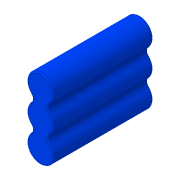
# Autodesk Inventor part: BatteryPack6600mAh
Saved by Autodesk Inventor 2017 (Build 210142000, 142)
## iProperties
Part Number: BatteryPack6600mAh
Material: Generisch
Document SubType Name: Modeling
Designer: Werkstatt
Density: 1 g/cm^3
Appearance: Vorgabe(1)
Author: Werkstatt
Autodesk Inventor part; units mm, degrees
ref_plane "YZ Plane" through (0, 0, 0) normal (1, 0, 0) x (0, 1, 0)
ref_plane "XZ Plane" through (0, 0, 0) normal (0, 1, 0) x (-1, 0, 0)
ref_plane "XY Plane" through (0, 0, 0) normal (0, 0, 1) x (1, 0, 0)
sketch "Skizze1" plane through (0, 0, 0) normal (0, 1, 0) x (-1, 0, 0)
  arc A0 (6.47, 11.83) -> (0, 27.45) centre (0, 18.3) ccw
  line L0 (9.15, 18.3) -> (9.15, 0) construction
  arc A1 (6.47, 11.83) -> (6.47, 6.47) centre (9.15, 9.15) ccw
  arc A2 (9.15, 0) -> (6.47, 6.47) centre (0, 0) ccw
  line L1 (0, 18.3) -> (0, 0) construction
  line L2 (0, 18.3) -> (0, 27.45) construction
  arc A3 (0, 27.45) -> (-6.47, 11.83) centre (0, 18.3) ccw
  arc A4 (-6.47, 6.47) -> (-6.47, 11.83) centre (-9.15, 9.15) ccw
  arc A5 (-6.47, 6.47) -> (-9.15, 0) centre (0, 0) ccw
  line L3 (9.15, 0) -> (-9.15, 0) construction
  line L4 (14.3464, 0) -> (-13.2665, 0) construction
  arc A6 (0, -27.45) -> (6.47, -11.83) centre (0, -18.3) ccw
  arc A7 (6.47, -6.47) -> (6.47, -11.83) centre (9.15, -9.15) ccw
  arc A8 (6.47, -6.47) -> (9.15, 0) centre (0, 0) ccw
  arc A9 (-6.47, -11.83) -> (-6.47, -6.47) centre (-9.15, -9.15) ccw
  arc A10 (-9.15, 0) -> (-6.47, -6.47) centre (0, 0) ccw
  arc A11 (-6.47, -11.83) -> (0, -27.45) centre (0, -18.3) ccw
  dimension "d1" = 18.3
  dimension "d3" = 9.15
  dimension "d5" = 9.15
  dimension "d6" = 9.15
  dimension "d7" = 9.15
  dimension "d8" = 3.79
  constraints: 25 point on circle, 12 centre point, 12 symmetric about line, 10 end point, 2 horizontal, 2 vertical, 1 coincident, 1 midpoint, 9 other
  measures "d1" distance of point (0, 0) L1.start
  measures "d3" horizontal distance of point (0, 0) A1.centre
  measures "d5" radius of A2
  measures "d6" radius of A0
  measures "d7" horizontal distance of point (0, 0) A1.centre
  measures "d8" radius of A1
extrude "Extrusion1" add sketch "Skizze1" along normal blind 69
fillet "Rundung1" radius 1 16 edges at (5.3599, 69, 9.15) (8.4535, 69, -3.5016) (5.3599, 69, -9.15) (-8.4535, 69, -21.8016) (-5.3599, 69, -9.15) (-8.4535, 69, 3.5016) (-5.3599, 69, 9.15) (8.4535, 69, 21.8016) (5.3599, 0, 9.15) (8.4535, 0, 3.5016) (5.3599, 0, -9.15) (-8.4535, 0, -21.8016) (-5.3599, 0, -9.15) (-8.4535, 0, 3.5016) (-5.3599, 0, 9.15) (-8.4535, 0, 21.8016)
